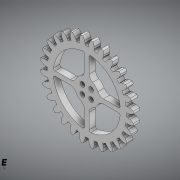
# Autodesk Inventor part: m2z28
Saved by Autodesk Inventor 2020 (Build 240168000, 168)
## iProperties
Created: 2019-12-19
Part Number: m2z28
Material: 一般
Document SubType Name: Modeling
Designer: hamaa
Density: 1 g/cm^3
Appearance: 既定
Author: hamaa
Autodesk Inventor part; units mm, degrees
(part 1 of 2)
ref_plane "YZ Plane" through (0, 0, 0) normal (1, 0, 0) x (0, 1, 0)
ref_plane "XZ Plane" through (0, 0, 0) normal (0, 1, 0) x (-1, 0, 0)
ref_plane "XY Plane" through (0, 0, 0) normal (0, 0, 1) x (1, 0, 0)
sketch "スケッチ1" plane through (0, 0, 0) normal (0, 0, 1) x (1, 0, 0)
  arc A0 (149.6341, 131.6283) -> (149.5837, 131.2892) centre (152.0661, 131.0939) ccw
  arc A1 (149.9967, 132.7811) -> (149.6341, 131.6283) centre (156.3128, 130.1609) ccw
  arc A2 (151.1315, 134.8845) -> (149.9967, 132.7811) centre (160.8866, 128.2635) ccw
  arc A3 (143.6803, 131.213) -> (143.7067, 130.8712) centre (146.1702, 131.2332) ccw
  arc A4 (143.7773, 132.4176) -> (143.6803, 131.213) centre (150.5181, 131.2686) ccw
  arc A5 (144.4157, 134.7208) -> (143.7773, 132.4176) centre (155.3994, 130.4365) ccw
  arc A6 (137.9682, 129.4833) -> (138.07, 129.156) centre (140.3912, 130.0571) ccw
  arc A7 (137.7948, 130.6793) -> (137.9682, 129.4833) centre (144.6222, 131.0591) ccw
  arc A8 (137.9046, 133.0668) -> (137.7948, 130.6793) centre (149.5663, 131.334) ccw
  arc A9 (132.7843, 126.5259) -> (132.9563, 126.2295) centre (135.0188, 127.6245) ccw
  arc A10 (132.349, 127.6534) -> (132.7843, 126.5259) centre (138.9208, 129.5428) ccw
  arc A11 (131.9248, 130.0054) -> (132.349, 127.6534) centre (143.6798, 130.9111) ccw
  arc A12 (128.3884, 122.4892) -> (128.6221, 122.2384) centre (130.3224, 124.0574) ccw
  arc A13 (127.7131, 123.4915) -> (128.3884, 122.4892) centre (133.6997, 126.7959) ccw
  arc A14 (126.7762, 125.6902) -> (127.7131, 123.4915) centre (138.0349, 129.1888) ccw
  arc A15 (125.0009, 117.5754) -> (125.2846, 117.383) centre (126.5375, 119.5348) ccw
  arc A16 (124.1196, 118.4024) -> (125.0009, 117.5754) centre (129.2208, 122.9561) ccw
  arc A17 (122.7169, 120.3375) -> (124.1196, 118.4024) centre (132.9148, 126.2537) ccw
  arc A18 (122.7918, 112.0311) -> (123.1112, 111.9066) centre (123.8539, 114.2832) ccw
  arc A19 (121.7486, 112.6412) -> (122.7918, 112.0311) centre (125.7086, 118.2159) ccw
  arc A20 (119.9505, 114.2156) -> (121.7486, 112.6412) centre (128.5762, 122.2528) ccw
  arc A21 (121.8719, 106.1342) -> (122.2109, 106.0839) centre (122.4062, 108.5662) ccw
  arc A22 (120.719, 106.4969) -> (121.8719, 106.1342) centre (123.3392, 112.813) ccw
  arc A23 (118.6156, 107.6317) -> (120.719, 106.4969) centre (125.2366, 117.3868) ccw
  arc A24 (122.2871, 100.1805) -> (122.6289, 100.2069) centre (122.2669, 102.6704) ccw
  arc A25 (121.0825, 100.2775) -> (122.2871, 100.1805) centre (122.2315, 107.0183) ccw
  arc A26 (118.7793, 100.9159) -> (121.0825, 100.2775) centre (123.0636, 111.8996) ccw
  arc A27 (124.0168, 94.4684) -> (124.3441, 94.5702) centre (123.443, 96.8914) ccw
  arc A28 (122.8208, 94.2949) -> (124.0168, 94.4684) centre (122.441, 101.1224) ccw
  arc A29 (120.4333, 94.4048) -> (122.8208, 94.2949) centre (122.1661, 106.0665) ccw
  arc A30 (126.9742, 89.2845) -> (127.2707, 89.4565) centre (125.8756, 91.519) ccw
  arc A31 (125.8467, 88.8492) -> (126.9742, 89.2845) centre (123.9573, 95.421) ccw
  arc A32 (123.4947, 88.425) -> (125.8467, 88.8492) centre (122.589, 100.1799) ccw
  arc A33 (131.0109, 84.8886) -> (131.2617, 85.1223) centre (129.4427, 86.8226) ccw
  arc A34 (130.0086, 84.2133) -> (131.0109, 84.8886) centre (126.7042, 90.1999) ccw
  arc A35 (127.8099, 83.2764) -> (130.0086, 84.2133) centre (124.3113, 94.5351) ccw
  arc A36 (135.9247, 81.5011) -> (136.1172, 81.7848) centre (133.9654, 83.0377) ccw
  arc A37 (135.0977, 80.6198) -> (135.9247, 81.5011) centre (130.544, 85.721) ccw
  arc A38 (133.1627, 79.2171) -> (135.0977, 80.6198) centre (127.2464, 89.415) ccw
  arc A39 (141.469, 79.292) -> (141.5935, 79.6114) centre (139.2169, 80.3541) ccw
  arc A40 (140.8589, 78.2488) -> (141.469, 79.292) centre (135.2842, 82.2087) ccw
  arc A41 (139.2845, 76.4506) -> (140.8589, 78.2488) centre (131.2473, 85.0764) ccw
  arc A42 (147.3659, 78.372) -> (147.4162, 78.7111) centre (144.9339, 78.9064) ccw
  arc A43 (147.0032, 77.2192) -> (147.3659, 78.372) centre (140.6871, 79.8394) ccw
  arc A44 (145.8684, 75.1158) -> (147.0032, 77.2192) centre (136.1133, 81.7368) ccw
  arc A45 (153.3196, 78.7873) -> (153.2932, 79.1291) centre (150.8297, 78.7671) ccw
  arc A46 (153.2226, 77.5827) -> (153.3196, 78.7873) centre (146.4818, 78.7317) ccw
  arc A47 (152.5843, 75.2795) -> (153.2226, 77.5827) centre (141.6005, 79.5638) ccw
  arc A48 (159.0317, 80.517) -> (158.9299, 80.8443) centre (156.6087, 79.9432) ccw
  arc A49 (159.2052, 79.321) -> (159.0317, 80.517) centre (152.3777, 78.9412) ccw
  arc A50 (159.0953, 76.9335) -> (159.2052, 79.321) centre (147.4336, 78.6663) ccw
  arc A51 (164.2156, 83.4744) -> (164.0436, 83.7708) centre (161.9811, 82.3758) ccw
  arc A52 (164.6509, 82.3469) -> (164.2156, 83.4744) centre (158.0791, 80.4575) ccw
  arc A53 (165.0751, 79.9949) -> (164.6509, 82.3469) centre (153.3202, 79.0892) ccw
  arc A54 (168.6116, 87.5111) -> (168.3778, 87.7619) centre (166.6775, 85.9429) ccw
  arc A55 (169.2868, 86.5088) -> (168.6116, 87.5111) centre (163.3002, 83.2044) ccw
  arc A56 (170.2237, 84.3101) -> (169.2868, 86.5088) centre (158.965, 80.8115) ccw
  arc A57 (171.999, 92.4249) -> (171.7153, 92.6173) centre (170.4624, 90.4655) ccw
  arc A58 (172.8803, 91.5979) -> (171.999, 92.4249) centre (167.7792, 87.0442) ccw
  arc A59 (174.283, 89.6628) -> (172.8803, 91.5979) centre (164.0851, 83.7466) ccw
  arc A60 (174.2081, 97.9692) -> (173.8887, 98.0937) centre (173.146, 95.7171) ccw
  arc A61 (175.2514, 97.3591) -> (174.2081, 97.9692) centre (171.2914, 91.7844) ccw
  arc A62 (177.0495, 95.7847) -> (175.2514, 97.3591) centre (168.4237, 87.7475) ccw
  arc A63 (175.1281, 103.8661) -> (174.789, 103.9164) centre (174.5937, 101.4341) ccw
  arc A64 (176.2809, 103.5034) -> (175.1281, 103.8661) centre (173.6607, 97.1873) ccw
  arc A65 (178.3843, 102.3686) -> (176.2809, 103.5034) centre (171.7633, 92.6135) ccw
  arc A66 (174.7128, 109.8198) -> (174.371, 109.7934) centre (174.733, 107.3299) ccw
  arc A67 (175.9175, 109.7228) -> (174.7128, 109.8198) centre (174.7684, 102.982) ccw
  arc A68 (178.2206, 109.0844) -> (175.9175, 109.7228) centre (173.9363, 98.1007) ccw
  arc A69 (172.9831, 115.5319) -> (172.6558, 115.4301) centre (173.5569, 113.1089) ccw
  arc A70 (174.1792, 115.7054) -> (172.9831, 115.5319) centre (174.5589, 108.8779) ccw
  arc A71 (176.5666, 115.5955) -> (174.1792, 115.7054) centre (174.8338, 103.9338) ccw
  arc A72 (170.0257, 120.7158) -> (169.7293, 120.5438) centre (171.1243, 118.4813) ccw
  arc A73 (171.1532, 121.1511) -> (170.0257, 120.7158) centre (173.0426, 114.5793) ccw
  arc A74 (173.5053, 121.5753) -> (171.1532, 121.1511) centre (174.4109, 109.8203) ccw
  arc A75 (165.989, 125.1117) -> (165.7382, 124.878) centre (167.5573, 123.1777) ccw
  arc A76 (166.9913, 125.787) -> (165.989, 125.1117) centre (170.2957, 119.8004) ccw
  arc A77 (169.19, 126.7239) -> (166.9913, 125.787) centre (172.6887, 115.4652) ccw
  arc A78 (161.0752, 128.4992) -> (160.8828, 128.2155) centre (163.0346, 126.9626) ccw
  arc A79 (161.9022, 129.3805) -> (161.0752, 128.4992) centre (166.4559, 124.2793) ccw
  arc A80 (163.8373, 130.7832) -> (161.9022, 129.3805) centre (169.7535, 120.5853) ccw
  arc A81 (155.5309, 130.7083) -> (155.4064, 130.3889) centre (157.7831, 129.6462) ccw
  arc A82 (156.141, 131.7515) -> (155.5309, 130.7083) centre (161.7157, 127.7915) ccw
  arc A83 (157.7155, 133.5497) -> (156.141, 131.7515) centre (165.7526, 124.9239) ccw
  arc A84 (147.4162, 131.2892) -> (147.3659, 131.6283) centre (144.9339, 131.0939) ccw
  arc A85 (147.3659, 131.6283) -> (147.0032, 132.7811) centre (140.6871, 130.1609) ccw
  arc A86 (147.0032, 132.7811) -> (145.8684, 134.8845) centre (136.1133, 128.2635) ccw
  arc A87 (141.5935, 130.3889) -> (141.469, 130.7083) centre (139.2169, 129.6462) ccw
  arc A88 (141.469, 130.7083) -> (140.8589, 131.7515) centre (135.2842, 127.7915) ccw
  arc A89 (140.8589, 131.7515) -> (139.2845, 133.5497) centre (131.2473, 124.9239) ccw
  arc A90 (136.1172, 128.2155) -> (135.9247, 128.4992) centre (133.9654, 126.9626) ccw
  arc A91 (135.9247, 128.4992) -> (135.0977, 129.3805) centre (130.544, 124.2793) ccw
  arc A92 (135.0977, 129.3805) -> (133.1627, 130.7832) centre (127.2464, 120.5853) ccw
  arc A93 (131.2617, 124.878) -> (131.0109, 125.1117) centre (129.4427, 123.1777) ccw
  arc A94 (131.0109, 125.1117) -> (130.0086, 125.787) centre (126.7042, 119.8004) ccw
  arc A95 (130.0086, 125.787) -> (127.8099, 126.7239) centre (124.3113, 115.4652) ccw
  arc A96 (127.2707, 120.5438) -> (126.9742, 120.7158) centre (125.8756, 118.4813) ccw
  arc A97 (126.9742, 120.7158) -> (125.8467, 121.1511) centre (123.9573, 114.5793) ccw
  arc A98 (125.8467, 121.1511) -> (123.4947, 121.5753) centre (122.589, 109.8203) ccw
  arc A99 (124.3441, 115.4301) -> (124.0168, 115.5319) centre (123.443, 113.1089) ccw
  arc A100 (124.0168, 115.5319) -> (122.8208, 115.7054) centre (122.441, 108.8779) ccw
  arc A101 (122.8208, 115.7054) -> (120.4333, 115.5955) centre (122.1661, 103.9338) ccw
  arc A102 (122.6289, 109.7934) -> (122.2871, 109.8198) centre (122.2669, 107.3299) ccw
  arc A103 (122.2871, 109.8198) -> (121.0825, 109.7228) centre (122.2315, 102.982) ccw
  arc A104 (121.0825, 109.7228) -> (118.7793, 109.0844) centre (123.0636, 98.1007) ccw
  arc A105 (122.2109, 103.9164) -> (121.8719, 103.8661) centre (122.4062, 101.4341) ccw
  arc A106 (121.8719, 103.8661) -> (120.719, 103.5034) centre (123.3392, 97.1873) ccw
  arc A107 (120.719, 103.5034) -> (118.6156, 102.3686) centre (125.2366, 92.6135) ccw
  arc A108 (123.1112, 98.0937) -> (122.7918, 97.9692) centre (123.8539, 95.7171) ccw
  arc A109 (122.7918, 97.9692) -> (121.7486, 97.3591) centre (125.7086, 91.7844) ccw
  arc A110 (121.7486, 97.3591) -> (119.9505, 95.7847) centre (128.5762, 87.7475) ccw
  arc A111 (125.2846, 92.6173) -> (125.0009, 92.4249) centre (126.5375, 90.4655) ccw
  arc A112 (125.0009, 92.4249) -> (124.1196, 91.5979) centre (129.2208, 87.0442) ccw
  arc A113 (124.1196, 91.5979) -> (122.7169, 89.6628) centre (132.9148, 83.7466) ccw
  arc A114 (128.6221, 87.7619) -> (128.3884, 87.5111) centre (130.3224, 85.9429) ccw
  arc A115 (128.3884, 87.5111) -> (127.7131, 86.5088) centre (133.6997, 83.2044) ccw
  arc A116 (127.7131, 86.5088) -> (126.7762, 84.3101) centre (138.0349, 80.8115) ccw
  arc A117 (132.9563, 83.7708) -> (132.7843, 83.4744) centre (135.0188, 82.3758) ccw
  arc A118 (132.7843, 83.4744) -> (132.349, 82.3469) centre (138.9208, 80.4575) ccw
  arc A119 (132.349, 82.3469) -> (131.9248, 79.9949) centre (143.6798, 79.0892) ccw
  arc A120 (138.07, 80.8443) -> (137.9682, 80.517) centre (140.3912, 79.9432) ccw
  arc A121 (137.9682, 80.517) -> (137.7948, 79.321) centre (144.6222, 78.9412) ccw
  arc A122 (137.7948, 79.321) -> (137.9046, 76.9335) centre (149.5663, 78.6663) ccw
  arc A123 (143.7067, 79.1291) -> (143.6803, 78.7873) centre (146.1702, 78.7671) ccw
  arc A124 (143.6803, 78.7873) -> (143.7773, 77.5827) centre (150.5181, 78.7317) ccw
  arc A125 (143.7773, 77.5827) -> (144.4157, 75.2795) centre (155.3994, 79.5638) ccw
  arc A126 (149.5837, 78.7111) -> (149.6341, 78.372) centre (152.0661, 78.9064) ccw
  arc A127 (149.6341, 78.372) -> (149.9967, 77.2192) centre (156.3128, 79.8394) ccw
  arc A128 (149.9967, 77.2192) -> (151.1315, 75.1158) centre (160.8866, 81.7368) ccw
  arc A129 (155.4064, 79.6114) -> (155.5309, 79.292) centre (157.7831, 80.3541) ccw
  arc A130 (155.5309, 79.292) -> (156.141, 78.2488) centre (161.7157, 82.2087) ccw
  arc A131 (156.141, 78.2488) -> (157.7155, 76.4506) centre (165.7526, 85.0764) ccw
  arc A132 (160.8828, 81.7848) -> (161.0752, 81.5011) centre (163.0346, 83.0377) ccw
  arc A133 (161.0752, 81.5011) -> (161.9022, 80.6198) centre (166.4559, 85.721) ccw
  arc A134 (161.9022, 80.6198) -> (163.8373, 79.2171) centre (169.7535, 89.415) ccw
  arc A135 (165.7382, 85.1223) -> (165.989, 84.8886) centre (167.5573, 86.8226) ccw
  arc A136 (165.989, 84.8886) -> (166.9913, 84.2133) centre (170.2957, 90.1999) ccw
  arc A137 (166.9913, 84.2133) -> (169.19, 83.2764) centre (172.6887, 94.5351) ccw
  arc A138 (169.7293, 89.4565) -> (170.0257, 89.2845) centre (171.1243, 91.519) ccw
  arc A139 (170.0257, 89.2845) -> (171.1532, 88.8492) centre (173.0426, 95.421) ccw
  arc A140 (171.1532, 88.8492) -> (173.5053, 88.425) centre (174.4109, 100.1799) ccw
  arc A141 (172.6558, 94.5702) -> (172.9831, 94.4684) centre (173.5569, 96.8914) ccw
  arc A142 (172.9831, 94.4684) -> (174.1792, 94.2949) centre (174.5589, 101.1224) ccw
  arc A143 (174.1792, 94.2949) -> (176.5666, 94.4048) centre (174.8338, 106.0665) ccw
  arc A144 (174.371, 100.2069) -> (174.7128, 100.1805) centre (174.733, 102.6704) ccw
  arc A145 (174.7128, 100.1805) -> (175.9175, 100.2775) centre (174.7684, 107.0183) ccw
  arc A146 (175.9175, 100.2775) -> (178.2206, 100.9159) centre (173.9363, 111.8996) ccw
  arc A147 (174.789, 106.0839) -> (175.1281, 106.1342) centre (174.5937, 108.5662) ccw
  arc A148 (175.1281, 106.1342) -> (176.2809, 106.4969) centre (173.6607, 112.813) ccw
  arc A149 (176.2809, 106.4969) -> (178.3843, 107.6317) centre (171.7633, 117.3868) ccw
  arc A150 (173.8887, 111.9066) -> (174.2081, 112.0311) centre (173.146, 114.2832) ccw
  arc A151 (174.2081, 112.0311) -> (175.2514, 112.6412) centre (171.2914, 118.2159) ccw
  arc A152 (175.2514, 112.6412) -> (177.0495, 114.2156) centre (168.4237, 122.2528) ccw
  arc A153 (171.7153, 117.383) -> (171.999, 117.5754) centre (170.4624, 119.5348) ccw
  arc A154 (171.999, 117.5754) -> (172.8803, 118.4024) centre (167.7792, 122.9561) ccw
  arc A155 (172.8803, 118.4024) -> (174.283, 120.3375) centre (164.0851, 126.2537) ccw
  arc A156 (168.3778, 122.2384) -> (168.6116, 122.4892) centre (166.6775, 124.0574) ccw
  arc A157 (168.6116, 122.4892) -> (169.2868, 123.4915) centre (163.3002, 126.7959) ccw
  arc A158 (169.2868, 123.4915) -> (170.2237, 125.6902) centre (158.965, 129.1888) ccw
  arc A159 (164.0436, 126.2295) -> (164.2156, 126.5259) centre (161.9811, 127.6245) ccw
  arc A160 (164.2156, 126.5259) -> (164.6509, 127.6534) centre (158.0791, 129.5428) ccw
  arc A161 (164.6509, 127.6534) -> (165.0751, 130.0054) centre (153.3202, 130.9111) ccw
  arc A162 (158.9299, 129.156) -> (159.0317, 129.4833) centre (156.6087, 130.0571) ccw
  arc A163 (159.0317, 129.4833) -> (159.2052, 130.6793) centre (152.3777, 131.0591) ccw
  arc A164 (159.2052, 130.6793) -> (159.0953, 133.0668) centre (147.4336, 131.334) ccw
  arc A165 (153.2932, 130.8712) -> (153.3196, 131.213) centre (150.8297, 131.2332) ccw
  arc A166 (153.3196, 131.213) -> (153.2226, 132.4176) centre (146.4818, 131.2686) ccw
  arc A167 (153.2226, 132.4176) -> (152.5843, 134.7208) centre (141.6005, 130.4365) ccw
  arc A168 (149.5503, 130.4785) -> (147.4496, 130.4785) centre (148.5, 105.0001) ccw
  arc A169 (143.8545, 130.0734) -> (141.8065, 129.606) centre (148.5, 105.0001) ccw
  arc A170 (138.3916, 128.4111) -> (136.499, 127.4996) centre (148.5, 105.0001) ccw
  arc A171 (133.4357, 125.5748) -> (131.7933, 124.2651) centre (148.5, 105.0001) ccw
  arc A172 (129.2351, 121.7068) -> (127.9253, 120.0645) centre (148.5, 105.0001) ccw
  arc A173 (126.0005, 117.0011) -> (125.089, 115.1085) centre (148.5, 105.0001) ccw
  arc A174 (123.8941, 111.6936) -> (123.4267, 109.6456) centre (148.5, 105.0001) ccw
  arc A175 (123.0216, 106.0505) -> (123.0216, 103.9498) centre (148.5, 105.0001) ccw
  arc A176 (123.4267, 100.3547) -> (123.8941, 98.3067) centre (148.5, 105.0001) ccw
  arc A177 (125.089, 94.8918) -> (126.0005, 92.9992) centre (148.5, 105.0001) ccw
  arc A178 (127.9253, 89.9358) -> (129.2351, 88.2935) centre (148.5, 105.0001) ccw
  arc A179 (131.7933, 85.7352) -> (133.4357, 84.4255) centre (148.5, 105.0001) ccw
  arc A180 (136.499, 82.5007) -> (138.3916, 81.5892) centre (148.5, 105.0001) ccw
  arc A181 (141.8065, 80.3943) -> (143.8545, 79.9269) centre (148.5, 105.0001) ccw
  arc A182 (147.4496, 79.5218) -> (149.5503, 79.5218) centre (148.5, 105.0001) ccw
  arc A183 (153.1454, 79.9269) -> (155.1934, 80.3943) centre (148.5, 105.0001) ccw
  arc A184 (158.6083, 81.5892) -> (160.5009, 82.5007) centre (148.5, 105.0001) ccw
  arc A185 (163.5643, 84.4255) -> (165.2066, 85.7352) centre (148.5, 105.0001) ccw
  arc A186 (167.7649, 88.2935) -> (169.0746, 89.9358) centre (148.5, 105.0001) ccw
  arc A187 (170.9994, 92.9992) -> (171.9109, 94.8918) centre (148.5, 105.0001) ccw
  arc A188 (173.1058, 98.3067) -> (173.5732, 100.3547) centre (148.5, 105.0001) ccw
  arc A189 (173.9783, 103.9498) -> (173.9783, 106.0505) centre (148.5, 105.0001) ccw
  arc A190 (173.5732, 109.6456) -> (173.1058, 111.6936) centre (148.5, 105.0001) ccw
  arc A191 (171.9109, 115.1085) -> (170.9994, 117.0011) centre (148.5, 105.0001) ccw
  arc A192 (169.0746, 120.0645) -> (167.7649, 121.7068) centre (148.5, 105.0001) ccw
  arc A193 (165.2066, 124.2651) -> (163.5643, 125.5748) centre (148.5, 105.0001) ccw
  arc A194 (160.5009, 127.4996) -> (158.6083, 128.4111) centre (148.5, 105.0001) ccw
  arc A195 (155.1934, 129.606) -> (153.1454, 130.0734) centre (148.5, 105.0001) ccw
  arc A196 (145.8684, 134.8845) -> (144.4157, 134.7208) centre (148.5, 105.0001) ccw
  arc A197 (139.2845, 133.5497) -> (137.9046, 133.0668) centre (148.5, 105.0001) ccw
  arc A198 (133.1627, 130.7832) -> (131.9248, 130.0054) centre (148.5, 105.0001) ccw
  arc A199 (127.8099, 126.7239) -> (126.7762, 125.6902) centre (148.5, 105.0001) ccw
  arc A200 (123.4947, 121.5753) -> (122.7169, 120.3375) centre (148.5, 105.0001) ccw
  arc A201 (120.4333, 115.5955) -> (119.9505, 114.2156) centre (148.5, 105.0001) ccw
  arc A202 (118.7793, 109.0844) -> (118.6156, 107.6317) centre (148.5, 105.0001) ccw
  arc A203 (118.6156, 102.3686) -> (118.7793, 100.9159) centre (148.5, 105.0001) ccw
  arc A204 (119.9505, 95.7847) -> (120.4333, 94.4048) centre (148.5, 105.0001) ccw
  arc A205 (122.7169, 89.6628) -> (123.4947, 88.425) centre (148.5, 105.0001) ccw
  arc A206 (126.7762, 84.3101) -> (127.8099, 83.2764) centre (148.5, 105.0001) ccw
  arc A207 (131.9248, 79.9949) -> (133.1627, 79.2171) centre (148.5, 105.0001) ccw
  arc A208 (137.9046, 76.9335) -> (139.2845, 76.4506) centre (148.5, 105.0001) ccw
  arc A209 (144.4157, 75.2795) -> (145.8684, 75.1158) centre (148.5, 105.0001) ccw
  arc A210 (151.1315, 75.1158) -> (152.5843, 75.2795) centre (148.5, 105.0001) ccw
  arc A211 (157.7155, 76.4506) -> (159.0953, 76.9335) centre (148.5, 105.0001) ccw
  arc A212 (163.8373, 79.2171) -> (165.0751, 79.9949) centre (148.5, 105.0001) ccw
  arc A213 (169.19, 83.2764) -> (170.2237, 84.3101) centre (148.5, 105.0001) ccw
  arc A214 (173.5053, 88.425) -> (174.283, 89.6628) centre (148.5, 105.0001) ccw
  arc A215 (176.5666, 94.4048) -> (177.0495, 95.7847) centre (148.5, 105.0001) ccw
  arc A216 (178.2206, 100.9159) -> (178.3843, 102.3686) centre (148.5, 105.0001) ccw
  arc A217 (178.3843, 107.6317) -> (178.2206, 109.0844) centre (148.5, 105.0001) ccw
  arc A218 (177.0495, 114.2156) -> (176.5666, 115.5955) centre (148.5, 105.0001) ccw
  arc A219 (174.283, 120.3375) -> (173.5053, 121.5753) centre (148.5, 105.0001) ccw
  arc A220 (170.2237, 125.6902) -> (169.19, 126.7239) centre (148.5, 105.0001) ccw
  arc A221 (165.0751, 130.0054) -> (163.8373, 130.7832) centre (148.5, 105.0001) ccw
  arc A222 (159.0953, 133.0668) -> (157.7155, 133.5497) centre (148.5, 105.0001) ccw
  arc A223 (152.5843, 134.7208) -> (151.1315, 134.8845) centre (148.5, 105.0001) ccw
  line L0 (149.5503, 130.4785) -> (149.5837, 131.2892)
  line L1 (143.8545, 130.0734) -> (143.7067, 130.8712)
  line L2 (138.3916, 128.4111) -> (138.07, 129.156)
  line L3 (133.4357, 125.5748) -> (132.9563, 126.2295)
  line L4 (129.2351, 121.7068) -> (128.6221, 122.2384)
  line L5 (126.0005, 117.0011) -> (125.2846, 117.383)
  line L6 (123.8941, 111.6936) -> (123.1112, 111.9066)
  line L7 (123.0216, 106.0505) -> (122.2109, 106.0839)
  line L8 (123.4267, 100.3547) -> (122.6289, 100.2069)
  line L9 (125.089, 94.8918) -> (124.3441, 94.5702)
  line L10 (127.9253, 89.9358) -> (127.2707, 89.4565)
  line L11 (131.7933, 85.7352) -> (131.2617, 85.1223)
  line L12 (136.499, 82.5007) -> (136.1172, 81.7848)
  line L13 (141.8065, 80.3943) -> (141.5935, 79.6114)
  line L14 (147.4496, 79.5218) -> (147.4162, 78.7111)
  line L15 (153.1454, 79.9269) -> (153.2932, 79.1291)
  line L16 (158.6083, 81.5892) -> (158.9299, 80.8443)
  line L17 (163.5643, 84.4255) -> (164.0436, 83.7708)
  line L18 (167.7649, 88.2935) -> (168.3778, 87.7619)
  line L19 (170.9994, 92.9992) -> (171.7153, 92.6173)
  line L20 (173.1058, 98.3067) -> (173.8887, 98.0937)
  line L21 (173.9783, 103.9498) -> (174.789, 103.9164)
  line L22 (173.5732, 109.6456) -> (174.371, 109.7934)
  line L23 (171.9109, 115.1085) -> (172.6558, 115.4301)
  line L24 (169.0746, 120.0645) -> (169.7293, 120.5438)
  line L25 (165.2066, 124.2651) -> (165.7382, 124.878)
  line L26 (160.5009, 127.4996) -> (160.8828, 128.2155)
  line L27 (155.1934, 129.606) -> (155.4064, 130.3889)
  line L28 (147.4496, 130.4785) -> (147.4162, 131.2892)
  line L29 (141.8065, 129.606) -> (141.5935, 130.3889)
  line L30 (136.499, 127.4996) -> (136.1172, 128.2155)
  line L31 (131.7933, 124.2651) -> (131.2617, 124.878)
  line L32 (127.9253, 120.0645) -> (127.2707, 120.5438)
  line L33 (125.089, 115.1085) -> (124.3441, 115.4301)
  line L34 (123.4267, 109.6456) -> (122.6289, 109.7934)
  line L35 (123.0216, 103.9498) -> (122.2109, 103.9164)
  line L36 (123.8941, 98.3067) -> (123.1112, 98.0937)
  line L37 (126.0005, 92.9992) -> (125.2846, 92.6173)
  line L38 (129.2351, 88.2935) -> (128.6221, 87.7619)
  line L39 (133.4357, 84.4255) -> (132.9563, 83.7708)
  line L40 (138.3916, 81.5892) -> (138.07, 80.8443)
  line L41 (143.8545, 79.9269) -> (143.7067, 79.1291)
  line L42 (149.5503, 79.5218) -> (149.5837, 78.7111)
  line L43 (155.1934, 80.3943) -> (155.4064, 79.6114)
  line L44 (160.5009, 82.5007) -> (160.8828, 81.7848)
  line L45 (165.2066, 85.7352) -> (165.7382, 85.1223)
  line L46 (169.0746, 89.9358) -> (169.7293, 89.4565)
  line L47 (171.9109, 94.8918) -> (172.6558, 94.5702)
  line L48 (173.5732, 100.3547) -> (174.371, 100.2069)
  line L49 (173.9783, 106.0505) -> (174.789, 106.0839)
  line L50 (173.1058, 111.6936) -> (173.8887, 111.9066)
  line L51 (170.9994, 117.0011) -> (171.7153, 117.383)
  line L52 (167.7649, 121.7068) -> (168.3778, 122.2384)
  line L53 (163.5643, 125.5748) -> (164.0436, 126.2295)
  line L54 (158.6083, 128.4111) -> (158.9299, 129.156)
  line L55 (153.1454, 130.0734) -> (153.2932, 130.8712)
  line L56 (116.5, 105) -> (180.5, 105)
  line L57 (148.5, 73) -> (148.5, 137)
  line L58 (198.5, 135.0001) -> (268.5, 135.0001)
  line L59 (198.5, 127.0001) -> (268.5, 127.0001)
  line L60 (198.5, 119.0001) -> (268.5, 119.0001)
  line L61 (198.5, 111.0001) -> (268.5, 111.0001)
  line L62 (198.5, 103.0001) -> (268.5, 103.0001)
  line L63 (198.5, 95.0001) -> (268.5, 95.0001)
  line L64 (198.5, 87.0001) -> (268.5, 87.0001)
  line L65 (198.5, 79.0001) -> (268.5, 79.0001)
  line L66 (198.5, 71.0001) -> (268.5, 71.0001)
  line L67 (198.5, 63.0001) -> (268.5, 63.0001)
  line L68 (198.5, 55.0001) -> (268.5, 55.0001)
  line L69 (198.5, 47.0001) -> (268.5, 47.0001)
  line L70 (198.5, 39.0001) -> (268.5, 39.0001)
  line L71 (198.5, 135.0001) -> (198.5, 39.0001)
  line L72 (268.5, 135.0001) -> (268.5, 39.0001)
  line L73 (233.5, 127.0001) -> (233.5, 39.0001)
  point P0 (0, 0)
  point P1 (204.5, 129)
  point P2 (207, 121)
  point P3 (207, 113)
  point P4 (204.5, 105)
  point P5 (207, 97)
  point P6 (202, 89)
  point P7 (204.5, 81)
  point P8 (204.5, 73)
  point P9 (204.5, 65)
  point P10 (207, 57)
  point P11 (207, 49)
  point P12 (204.5, 41)
  point P13 (234.5, 121)
  point P14 (249.5, 113)
  point P15 (250.75, 105)
  point P16 (247, 97)
  point P17 (249.5, 89)
  point P18 (243.25, 81)
  point P19 (249.5, 73)
  point P20 (249.5, 65)
  point P21 (244.5, 57)
  point P22 (252, 49)
  point P23 (252, 41)
  point P24 (149.5, 150.5)
  point P25 (149.5, 144.5)
  point P26 (165.6875, 150.5)
  point P27 (168.875, 144.5)
  constraints: 336 point on circle, 168 centre point, 165 equal radius, 144 end point, 112 tangent, 41 parallel, 30 horizontal, 16 perpendicular, 2 horizontal alignment, 2 midpoint, 2 vertical alignment, 219 other
extrude "押し出し1" add sketch "スケッチ1" along normal blind 4 contours A1 A2 A223 A167 A166 A165 L55 A195 L27 A81 A82 A83 A222 A164 A163 A162 L54 A194 L26 A78 A79 A80 A221 A161 A160 A159 L53 A193 L25 A75 A76 A77 A220 A158 A157 A156 L52 A192 L24 A72 A73 A74 A219 A155 A154 A153 L51 A191 L23 A69 A70 A71 A218 A152 A151 A150 L50 A190 L22 A66 A67 A68 A217 A149 A148 A147 L49 A189 L56 L57 A168 L0 A0 | L57 L56 A175 L7 A21 A22 A23 A202 A104 A103 A102 L34 A174 L6 A18 A19 A20 A201 A101 A100 A99 L33 A173 L5 A15 A16 A17 A200 A98 A97 A96 L32 A172 L4 A12 A13 A14 A199 A95 A94 A93 L31 A171 L3 A9 A10 A11 A198 A92 A91 A90 L30 A170 L2 A6 A7 A8 A197 A89 A88 A87 L29 A169 L1 A3 A4 A5 A196 A86 A85 A84 L28 A168 | L57 A182 L14 A42 A43 A44 A209 A125 A124 A123 L41 A181 L13 A39 A40 A41 A208 A122 A121 A120 L40 A180 L12 A36 A37 A38 A207 A119 A118 A117 L39 A179 L11 A33 A34 A35 A206 A116 A115 A114 L38 A178 L10 A30 A31 A32 A205 A113 A112 A111 L37 A177 L9 A27 A28 A29 A204 A110 A109 A108 L36 A176 L8 A24 A25 A26 A203 A107 A106 A105 L35 A175 L56 | L56 A189 L21 A63 A64 A65 A216 A146 A145 A144 L48 A188 L20 A60 A61 A62 A215 A143 A142 A141 L47 A187 L19 A57 A58 A59 A214 A140 A139 A138 L46 A186 L18 A54 A55 A56 A213 A137 A136 A135 L45 A185 L17 A51 A52 A53 A212 A134 A133 A132 L44 A184 L16 A48 A49 A50 A211 A131 A130 A129 L43 A183 L15 A45 A46 A47 A210 A128 A127 A126 L42 A182 L57
sketch "スケッチ2" plane through (0, 0, 4) normal (0, 0, 1) x (1, 0, 0)
  arc A0 (147.4162, 131.2892) -> (147.3659, 131.6283) centre (144.9339, 131.0939) ccw projected
  arc A1 (147.3659, 131.6283) -> (147.0032, 132.7811) centre (140.6871, 130.1609) ccw projected
  arc A2 (147.0032, 132.7811) -> (145.8684, 134.8845) centre (136.1133, 128.2635) ccw projected
  arc A3 (145.8684, 134.8845) -> (144.4157, 134.7208) centre (148.5, 105.0001) ccw projected
  arc A4 (144.4157, 134.7208) -> (143.7773, 132.4176) centre (155.3994, 130.4365) ccw projected
  arc A5 (143.7773, 132.4176) -> (143.6803, 131.213) centre (150.5181, 131.2686) ccw projected
  arc A6 (143.6803, 131.213) -> (143.7067, 130.8712) centre (146.1702, 131.2332) ccw projected
  line L0 (143.7067, 130.8712) -> (143.8545, 130.0734) projected
  arc A7 (143.8545, 130.0734) -> (141.8065, 129.606) centre (148.5, 105.0001) ccw projected
  line L1 (141.8065, 129.606) -> (141.5935, 130.3889) projected
  arc A8 (141.5935, 130.3889) -> (141.469, 130.7083) centre (139.2169, 129.6462) ccw projected
  arc A9 (141.469, 130.7083) -> (140.8589, 131.7515) centre (135.2842, 127.7915) ccw projected
  arc A10 (140.8589, 131.7515) -> (139.2845, 133.5497) centre (131.2473, 124.9239) ccw projected
  arc A11 (139.2845, 133.5497) -> (137.9046, 133.0668) centre (148.5, 105.0001) ccw projected
  arc A12 (137.9046, 133.0668) -> (137.7948, 130.6793) centre (149.5663, 131.334) ccw projected
  arc A13 (137.7948, 130.6793) -> (137.9682, 129.4833) centre (144.6222, 131.0591) ccw projected
  arc A14 (137.9682, 129.4833) -> (138.07, 129.156) centre (140.3912, 130.0571) ccw projected
  line L2 (138.07, 129.156) -> (138.3916, 128.4111) projected
  arc A15 (138.3916, 128.4111) -> (136.499, 127.4996) centre (148.5, 105.0001) ccw projected
  line L3 (136.499, 127.4996) -> (136.1172, 128.2155) projected
  arc A16 (136.1172, 128.2155) -> (135.9247, 128.4992) centre (133.9654, 126.9626) ccw projected
  arc A17 (135.9247, 128.4992) -> (135.0977, 129.3805) centre (130.544, 124.2793) ccw projected
  arc A18 (135.0977, 129.3805) -> (133.1627, 130.7832) centre (127.2464, 120.5853) ccw projected
  arc A19 (133.1627, 130.7832) -> (131.9248, 130.0054) centre (148.5, 105.0001) ccw projected
  arc A20 (131.9248, 130.0054) -> (132.349, 127.6534) centre (143.6798, 130.9111) ccw projected
  arc A21 (132.349, 127.6534) -> (132.7843, 126.5259) centre (138.9208, 129.5428) ccw projected
  arc A22 (132.7843, 126.5259) -> (132.9563, 126.2295) centre (135.0188, 127.6245) ccw projected
  line L4 (132.9563, 126.2295) -> (133.4357, 125.5748) projected
  arc A23 (133.4357, 125.5748) -> (131.7933, 124.2651) centre (148.5, 105.0001) ccw projected
  line L5 (131.7933, 124.2651) -> (131.2617, 124.878) projected
  arc A24 (131.2617, 124.878) -> (131.0109, 125.1117) centre (129.4427, 123.1777) ccw projected
  arc A25 (131.0109, 125.1117) -> (130.0086, 125.787) centre (126.7042, 119.8004) ccw projected
  arc A26 (130.0086, 125.787) -> (127.8099, 126.7239) centre (124.3113, 115.4652) ccw projected
  arc A27 (127.8099, 126.7239) -> (126.7762, 125.6902) centre (148.5, 105.0001) ccw projected
  arc A28 (126.7762, 125.6902) -> (127.7131, 123.4915) centre (138.0349, 129.1888) ccw projected
  arc A29 (127.7131, 123.4915) -> (128.3884, 122.4892) centre (133.6997, 126.7959) ccw projected
  arc A30 (128.3884, 122.4892) -> (128.6221, 122.2384) centre (130.3224, 124.0574) ccw projected
  line L6 (128.6221, 122.2384) -> (129.2351, 121.7068) projected
  arc A31 (129.2351, 121.7068) -> (127.9253, 120.0645) centre (148.5, 105.0001) ccw projected
  line L7 (127.9253, 120.0645) -> (127.2707, 120.5438) projected
  arc A32 (127.2707, 120.5438) -> (126.9742, 120.7158) centre (125.8756, 118.4813) ccw projected
  arc A33 (126.9742, 120.7158) -> (125.8467, 121.1511) centre (123.9573, 114.5793) ccw projected
  arc A34 (125.8467, 121.1511) -> (123.4947, 121.5753) centre (122.589, 109.8203) ccw projected
  arc A35 (123.4947, 121.5753) -> (122.7169, 120.3375) centre (148.5, 105.0001) ccw projected
  arc A36 (122.7169, 120.3375) -> (124.1196, 118.4024) centre (132.9148, 126.2537) ccw projected
  arc A37 (124.1196, 118.4024) -> (125.0009, 117.5754) centre (129.2208, 122.9561) ccw projected
  arc A38 (125.0009, 117.5754) -> (125.2846, 117.383) centre (126.5375, 119.5348) ccw projected
  line L8 (125.2846, 117.383) -> (126.0005, 117.0011) projected
  arc A39 (126.0005, 117.0011) -> (125.089, 115.1085) centre (148.5, 105.0001) ccw projected
  line L9 (125.089, 115.1085) -> (124.3441, 115.4301) projected
  arc A40 (124.3441, 115.4301) -> (124.0168, 115.5319) centre (123.443, 113.1089) ccw projected
  arc A41 (124.0168, 115.5319) -> (122.8208, 115.7054) centre (122.441, 108.8779) ccw projected
  arc A42 (122.8208, 115.7054) -> (120.4333, 115.5955) centre (122.1661, 103.9338) ccw projected
  arc A43 (120.4333, 115.5955) -> (119.9505, 114.2156) centre (148.5, 105.0001) ccw projected
  arc A44 (119.9505, 114.2156) -> (121.7486, 112.6412) centre (128.5762, 122.2528) ccw projected
  arc A45 (121.7486, 112.6412) -> (122.7918, 112.0311) centre (125.7086, 118.2159) ccw projected
  arc A46 (122.7918, 112.0311) -> (123.1112, 111.9066) centre (123.8539, 114.2832) ccw projected
  line L10 (123.1112, 111.9066) -> (123.8941, 111.6936) projected
  arc A47 (123.8941, 111.6936) -> (123.4267, 109.6456) centre (148.5, 105.0001) ccw projected
  line L11 (123.4267, 109.6456) -> (122.6289, 109.7934) projected
  arc A48 (122.6289, 109.7934) -> (122.2871, 109.8198) centre (122.2669, 107.3299) ccw projected
  arc A49 (122.2871, 109.8198) -> (121.0825, 109.7228) centre (122.2315, 102.982) ccw projected
  arc A50 (121.0825, 109.7228) -> (118.7793, 109.0844) centre (123.0636, 98.1007) ccw projected
  arc A51 (118.7793, 109.0844) -> (118.6156, 107.6317) centre (148.5, 105.0001) ccw projected
  arc A52 (118.6156, 107.6317) -> (120.719, 106.4969) centre (125.2366, 117.3868) ccw projected
  arc A53 (120.719, 106.4969) -> (121.8719, 106.1342) centre (123.3392, 112.813) ccw projected
  arc A54 (121.8719, 106.1342) -> (122.2109, 106.0839) centre (122.4062, 108.5662) ccw projected
  line L12 (122.2109, 106.0839) -> (123.0216, 106.0505) projected
  arc A55 (123.0216, 106.0505) -> (123.0216, 103.9498) centre (148.5, 105.0001) ccw projected
  line L13 (123.0216, 103.9498) -> (122.2109, 103.9164) projected
  arc A56 (122.2109, 103.9164) -> (121.8719, 103.8661) centre (122.4062, 101.4341) ccw projected
  arc A57 (121.8719, 103.8661) -> (120.719, 103.5034) centre (123.3392, 97.1873) ccw projected
  arc A58 (120.719, 103.5034) -> (118.6156, 102.3686) centre (125.2366, 92.6135) ccw projected
  arc A59 (118.6156, 102.3686) -> (118.7793, 100.9159) centre (148.5, 105.0001) ccw projected
  arc A60 (118.7793, 100.9159) -> (121.0825, 100.2775) centre (123.0636, 111.8996) ccw projected
  arc A61 (121.0825, 100.2775) -> (122.2871, 100.1805) centre (122.2315, 107.0183) ccw projected
  arc A62 (122.2871, 100.1805) -> (122.6289, 100.2069) centre (122.2669, 102.6704) ccw projected
  line L14 (122.6289, 100.2069) -> (123.4267, 100.3547) projected
  arc A63 (123.4267, 100.3547) -> (123.8941, 98.3067) centre (148.5, 105.0001) ccw projected
  line L15 (123.8941, 98.3067) -> (123.1112, 98.0937) projected
  arc A64 (123.1112, 98.0937) -> (122.7918, 97.9692) centre (123.8539, 95.7171) ccw projected
  arc A65 (122.7918, 97.9692) -> (121.7486, 97.3591) centre (125.7086, 91.7844) ccw projected
  arc A66 (121.7486, 97.3591) -> (119.9505, 95.7847) centre (128.5762, 87.7475) ccw projected
  arc A67 (119.9505, 95.7847) -> (120.4333, 94.4048) centre (148.5, 105.0001) ccw projected
  arc A68 (120.4333, 94.4048) -> (122.8208, 94.2949) centre (122.1661, 106.0665) ccw projected
  arc A69 (122.8208, 94.2949) -> (124.0168, 94.4684) centre (122.441, 101.1224) ccw projected
  arc A70 (124.0168, 94.4684) -> (124.3441, 94.5702) centre (123.443, 96.8914) ccw projected
  line L16 (124.3441, 94.5702) -> (125.089, 94.8918) projected
  arc A71 (125.089, 94.8918) -> (126.0005, 92.9992) centre (148.5, 105.0001) ccw projected
  line L17 (126.0005, 92.9992) -> (125.2846, 92.6173) projected
  arc A72 (125.2846, 92.6173) -> (125.0009, 92.4249) centre (126.5375, 90.4655) ccw projected
  arc A73 (125.0009, 92.4249) -> (124.1196, 91.5979) centre (129.2208, 87.0442) ccw projected
  arc A74 (124.1196, 91.5979) -> (122.7169, 89.6628) centre (132.9148, 83.7466) ccw projected
  arc A75 (122.7169, 89.6628) -> (123.4947, 88.425) centre (148.5, 105.0001) ccw projected
  arc A76 (123.4947, 88.425) -> (125.8467, 88.8492) centre (122.589, 100.1799) ccw projected
  arc A77 (125.8467, 88.8492) -> (126.9742, 89.2845) centre (123.9573, 95.421) ccw projected
  arc A78 (126.9742, 89.2845) -> (127.2707, 89.4565) centre (125.8756, 91.519) ccw projected
  line L18 (127.2707, 89.4565) -> (127.9253, 89.9358) projected
  arc A79 (127.9253, 89.9358) -> (129.2351, 88.2935) centre (148.5, 105.0001) ccw projected
  line L19 (129.2351, 88.2935) -> (128.6221, 87.7619) projected
  arc A80 (128.6221, 87.7619) -> (128.3884, 87.5111) centre (130.3224, 85.9429) ccw projected
  arc A81 (128.3884, 87.5111) -> (127.7131, 86.5088) centre (133.6997, 83.2044) ccw projected
  arc A82 (127.7131, 86.5088) -> (126.7762, 84.3101) centre (138.0349, 80.8115) ccw projected
  arc A83 (126.7762, 84.3101) -> (127.8099, 83.2764) centre (148.5, 105.0001) ccw projected
  arc A84 (127.8099, 83.2764) -> (130.0086, 84.2133) centre (124.3113, 94.5351) ccw projected
  arc A85 (130.0086, 84.2133) -> (131.0109, 84.8886) centre (126.7042, 90.1999) ccw projected
  arc A86 (131.0109, 84.8886) -> (131.2617, 85.1223) centre (129.4427, 86.8226) ccw projected
  line L20 (131.2617, 85.1223) -> (131.7933, 85.7352) projected
  arc A87 (131.7933, 85.7352) -> (133.4357, 84.4255) centre (148.5, 105.0001) ccw projected
  line L21 (133.4357, 84.4255) -> (132.9563, 83.7708) projected
  arc A88 (132.9563, 83.7708) -> (132.7843, 83.4744) centre (135.0188, 82.3758) ccw projected
  arc A89 (132.7843, 83.4744) -> (132.349, 82.3469) centre (138.9208, 80.4575) ccw projected
  arc A90 (132.349, 82.3469) -> (131.9248, 79.9949) centre (143.6798, 79.0892) ccw projected
  arc A91 (131.9248, 79.9949) -> (133.1627, 79.2171) centre (148.5, 105.0001) ccw projected
  arc A92 (133.1627, 79.2171) -> (135.0977, 80.6198) centre (127.2464, 89.415) ccw projected
  arc A93 (135.0977, 80.6198) -> (135.9247, 81.5011) centre (130.544, 85.721) ccw projected
  arc A94 (135.9247, 81.5011) -> (136.1172, 81.7848) centre (133.9654, 83.0377) ccw projected
  line L22 (136.1172, 81.7848) -> (136.499, 82.5007) projected
  arc A95 (136.499, 82.5007) -> (138.3916, 81.5892) centre (148.5, 105.0001) ccw projected
  line L23 (138.3916, 81.5892) -> (138.07, 80.8443) projected
  arc A96 (138.07, 80.8443) -> (137.9682, 80.517) centre (140.3912, 79.9432) ccw projected
  arc A97 (137.9682, 80.517) -> (137.7948, 79.321) centre (144.6222, 78.9412) ccw projected
  arc A98 (137.7948, 79.321) -> (137.9046, 76.9335) centre (149.5663, 78.6663) ccw projected
  arc A99 (137.9046, 76.9335) -> (139.2845, 76.4506) centre (148.5, 105.0001) ccw projected
  arc A100 (139.2845, 76.4506) -> (140.8589, 78.2488) centre (131.2473, 85.0764) ccw projected
  arc A101 (140.8589, 78.2488) -> (141.469, 79.292) centre (135.2842, 82.2087) ccw projected
  arc A102 (141.469, 79.292) -> (141.5935, 79.6114) centre (139.2169, 80.3541) ccw projected
  line L24 (141.5935, 79.6114) -> (141.8065, 80.3943) projected
  arc A103 (141.8065, 80.3943) -> (143.8545, 79.9269) centre (148.5, 105.0001) ccw projected
  line L25 (143.8545, 79.9269) -> (143.7067, 79.1291) projected
  arc A104 (143.7067, 79.1291) -> (143.6803, 78.7873) centre (146.1702, 78.7671) ccw projected
  arc A105 (143.6803, 78.7873) -> (143.7773, 77.5827) centre (150.5181, 78.7317) ccw projected
  arc A106 (143.7773, 77.5827) -> (144.4157, 75.2795) centre (155.3994, 79.5638) ccw projected
  arc A107 (144.4157, 75.2795) -> (145.8684, 75.1158) centre (148.5, 105.0001) ccw projected
  arc A108 (145.8684, 75.1158) -> (147.0032, 77.2192) centre (136.1133, 81.7368) ccw projected
  arc A109 (147.0032, 77.2192) -> (147.3659, 78.372) centre (140.6871, 79.8394) ccw projected
  arc A110 (147.3659, 78.372) -> (147.4162, 78.7111) centre (144.9339, 78.9064) ccw projected
  line L26 (147.4162, 78.7111) -> (147.4496, 79.5218) projected
  arc A111 (147.4496, 79.5218) -> (149.5503, 79.5218) centre (148.5, 105.0001) ccw projected
  line L27 (149.5503, 79.5218) -> (149.5837, 78.7111) projected
  arc A112 (149.5837, 78.7111) -> (149.6341, 78.372) centre (152.0661, 78.9064) ccw projected
  arc A113 (149.6341, 78.372) -> (149.9967, 77.2192) centre (156.3128, 79.8394) ccw projected
  arc A114 (149.9967, 77.2192) -> (151.1315, 75.1158) centre (160.8866, 81.7368) ccw projected
  arc A115 (151.1315, 75.1158) -> (152.5843, 75.2795) centre (148.5, 105.0001) ccw projected
  arc A116 (152.5843, 75.2795) -> (153.2226, 77.5827) centre (141.6005, 79.5638) ccw projected
  arc A117 (153.2226, 77.5827) -> (153.3196, 78.7873) centre (146.4818, 78.7317) ccw projected
  arc A118 (153.3196, 78.7873) -> (153.2932, 79.1291) centre (150.8297, 78.7671) ccw projected
  line L28 (153.2932, 79.1291) -> (153.1454, 79.9269) projected
  arc A119 (153.1454, 79.9269) -> (155.1934, 80.3943) centre (148.5, 105.0001) ccw projected
  line L29 (155.1934, 80.3943) -> (155.4064, 79.6114) projected
  arc A120 (155.4064, 79.6114) -> (155.5309, 79.292) centre (157.7831, 80.3541) ccw projected
  arc A121 (155.5309, 79.292) -> (156.141, 78.2488) centre (161.7157, 82.2087) ccw projected
  arc A122 (156.141, 78.2488) -> (157.7155, 76.4506) centre (165.7526, 85.0764) ccw projected
  arc A123 (157.7155, 76.4506) -> (159.0953, 76.9335) centre (148.5, 105.0001) ccw projected
  arc A124 (159.0953, 76.9335) -> (159.2052, 79.321) centre (147.4336, 78.6663) ccw projected
  arc A125 (159.2052, 79.321) -> (159.0317, 80.517) centre (152.3777, 78.9412) ccw projected
  arc A126 (159.0317, 80.517) -> (158.9299, 80.8443) centre (156.6087, 79.9432) ccw projected
  line L30 (158.9299, 80.8443) -> (158.6083, 81.5892) projected
  arc A127 (158.6083, 81.5892) -> (160.5009, 82.5007) centre (148.5, 105.0001) ccw projected
  line L31 (160.5009, 82.5007) -> (160.8828, 81.7848) projected
  arc A128 (160.8828, 81.7848) -> (161.0752, 81.5011) centre (163.0346, 83.0377) ccw projected
  arc A129 (161.0752, 81.5011) -> (161.9022, 80.6198) centre (166.4559, 85.721) ccw projected
  arc A130 (161.9022, 80.6198) -> (163.8373, 79.2171) centre (169.7535, 89.415) ccw projected
  arc A131 (163.8373, 79.2171) -> (165.0751, 79.9949) centre (148.5, 105.0001) ccw projected
  arc A132 (165.0751, 79.9949) -> (164.6509, 82.3469) centre (153.3202, 79.0892) ccw projected
  arc A133 (164.6509, 82.3469) -> (164.2156, 83.4744) centre (158.0791, 80.4575) ccw projected
  arc A134 (164.2156, 83.4744) -> (164.0436, 83.7708) centre (161.9811, 82.3758) ccw projected
  line L32 (164.0436, 83.7708) -> (163.5643, 84.4255) projected
  arc A135 (163.5643, 84.4255) -> (165.2066, 85.7352) centre (148.5, 105.0001) ccw projected
  line L33 (165.2066, 85.7352) -> (165.7382, 85.1223) projected
  arc A136 (165.7382, 85.1223) -> (165.989, 84.8886) centre (167.5573, 86.8226) ccw projected
  arc A137 (165.989, 84.8886) -> (166.9913, 84.2133) centre (170.2957, 90.1999) ccw projected
  arc A138 (166.9913, 84.2133) -> (169.19, 83.2764) centre (172.6887, 94.5351) ccw projected
  arc A139 (169.19, 83.2764) -> (170.2237, 84.3101) centre (148.5, 105.0001) ccw projected
  arc A140 (170.2237, 84.3101) -> (169.2868, 86.5088) centre (158.965, 80.8115) ccw projected
  arc A141 (169.2868, 86.5088) -> (168.6116, 87.5111) centre (163.3002, 83.2044) ccw projected
  arc A142 (168.6116, 87.5111) -> (168.3778, 87.7619) centre (166.6775, 85.9429) ccw projected
  line L34 (168.3778, 87.7619) -> (167.7649, 88.2935) projected
  arc A143 (167.7649, 88.2935) -> (169.0746, 89.9358) centre (148.5, 105.0001) ccw projected
  line L35 (169.0746, 89.9358) -> (169.7293, 89.4565) projected
  arc A144 (169.7293, 89.4565) -> (170.0257, 89.2845) centre (171.1243, 91.519) ccw projected
  arc A145 (170.0257, 89.2845) -> (171.1532, 88.8492) centre (173.0426, 95.421) ccw projected
  arc A146 (171.1532, 88.8492) -> (173.5053, 88.425) centre (174.4109, 100.1799) ccw projected
  arc A147 (173.5053, 88.425) -> (174.283, 89.6628) centre (148.5, 105.0001) ccw projected
  arc A148 (174.283, 89.6628) -> (172.8803, 91.5979) centre (164.0851, 83.7466) ccw projected
  arc A149 (172.8803, 91.5979) -> (171.999, 92.4249) centre (167.7792, 87.0442) ccw projected
  arc A150 (171.999, 92.4249) -> (171.7153, 92.6173) centre (170.4624, 90.4655) ccw projected
  line L36 (171.7153, 92.6173) -> (170.9994, 92.9992) projected
  arc A151 (170.9994, 92.9992) -> (171.9109, 94.8918) centre (148.5, 105.0001) ccw projected
  line L37 (171.9109, 94.8918) -> (172.6558, 94.5702) projected
  arc A152 (172.6558, 94.5702) -> (172.9831, 94.4684) centre (173.5569, 96.8914) ccw projected
  arc A153 (172.9831, 94.4684) -> (174.1792, 94.2949) centre (174.5589, 101.1224) ccw projected
  arc A154 (174.1792, 94.2949) -> (176.5666, 94.4048) centre (174.8338, 106.0665) ccw projected
  arc A155 (176.5666, 94.4048) -> (177.0495, 95.7847) centre (148.5, 105.0001) ccw projected
  arc A156 (177.0495, 95.7847) -> (175.2514, 97.3591) centre (168.4237, 87.7475) ccw projected
  arc A157 (175.2514, 97.3591) -> (174.2081, 97.9692) centre (171.2914, 91.7844) ccw projected
  arc A158 (174.2081, 97.9692) -> (173.8887, 98.0937) centre (173.146, 95.7171) ccw projected
  line L38 (173.8887, 98.0937) -> (173.1058, 98.3067) projected
  arc A159 (173.1058, 98.3067) -> (173.5732, 100.3547) centre (148.5, 105.0001) ccw projected
  line L39 (173.5732, 100.3547) -> (174.371, 100.2069) projected
  arc A160 (174.371, 100.2069) -> (174.7128, 100.1805) centre (174.733, 102.6704) ccw projected
  arc A161 (174.7128, 100.1805) -> (175.9175, 100.2775) centre (174.7684, 107.0183) ccw projected
  arc A162 (175.9175, 100.2775) -> (178.2206, 100.9159) centre (173.9363, 111.8996) ccw projected
  arc A163 (178.2206, 100.9159) -> (178.3843, 102.3686) centre (148.5, 105.0001) ccw projected
  arc A164 (178.3843, 102.3686) -> (176.2809, 103.5034) centre (171.7633, 92.6135) ccw projected
  arc A165 (176.2809, 103.5034) -> (175.1281, 103.8661) centre (173.6607, 97.1873) ccw projected
  arc A166 (175.1281, 103.8661) -> (174.789, 103.9164) centre (174.5937, 101.4341) ccw projected
  line L40 (174.789, 103.9164) -> (173.9783, 103.9498) projected
  arc A167 (173.9783, 103.9498) -> (173.9783, 106.0505) centre (148.5, 105.0001) ccw projected
  line L41 (173.9783, 106.0505) -> (174.789, 106.0839) projected
  arc A168 (174.789, 106.0839) -> (175.1281, 106.1342) centre (174.5937, 108.5662) ccw projected
  arc A169 (175.1281, 106.1342) -> (176.2809, 106.4969) centre (173.6607, 112.813) ccw projected
  arc A170 (176.2809, 106.4969) -> (178.3843, 107.6317) centre (171.7633, 117.3868) ccw projected
  arc A171 (178.3843, 107.6317) -> (178.2206, 109.0844) centre (148.5, 105.0001) ccw projected
  arc A172 (178.2206, 109.0844) -> (175.9175, 109.7228) centre (173.9363, 98.1007) ccw projected
  arc A173 (175.9175, 109.7228) -> (174.7128, 109.8198) centre (174.7684, 102.982) ccw projected
  arc A174 (174.7128, 109.8198) -> (174.371, 109.7934) centre (174.733, 107.3299) ccw projected
  line L42 (174.371, 109.7934) -> (173.5732, 109.6456) projected
  arc A175 (173.5732, 109.6456) -> (173.1058, 111.6936) centre (148.5, 105.0001) ccw projected
  line L43 (173.1058, 111.6936) -> (173.8887, 111.9066) projected
  arc A176 (173.8887, 111.9066) -> (174.2081, 112.0311) centre (173.146, 114.2832) ccw projected
  arc A177 (174.2081, 112.0311) -> (175.2514, 112.6412) centre (171.2914, 118.2159) ccw projected
  arc A178 (175.2514, 112.6412) -> (177.0495, 114.2156) centre (168.4237, 122.2528) ccw projected
  arc A179 (177.0495, 114.2156) -> (176.5666, 115.5955) centre (148.5, 105.0001) ccw projected
  arc A180 (176.5666, 115.5955) -> (174.1792, 115.7054) centre (174.8338, 103.9338) ccw projected
  arc A181 (174.1792, 115.7054) -> (172.9831, 115.5319) centre (174.5589, 108.8779) ccw projected
  arc A182 (172.9831, 115.5319) -> (172.6558, 115.4301) centre (173.5569, 113.1089) ccw projected
  line L44 (172.6558, 115.4301) -> (171.9109, 115.1085) projected
  arc A183 (171.9109, 115.1085) -> (170.9994, 117.0011) centre (148.5, 105.0001) ccw projected
  line L45 (170.9994, 117.0011) -> (171.7153, 117.383) projected
  arc A184 (171.7153, 117.383) -> (171.999, 117.5754) centre (170.4624, 119.5348) ccw projected
  arc A185 (171.999, 117.5754) -> (172.8803, 118.4024) centre (167.7792, 122.9561) ccw projected
  arc A186 (172.8803, 118.4024) -> (174.283, 120.3375) centre (164.0851, 126.2537) ccw projected
  arc A187 (174.283, 120.3375) -> (173.5053, 121.5753) centre (148.5, 105.0001) ccw projected
  arc A188 (173.5053, 121.5753) -> (171.1532, 121.1511) centre (174.4109, 109.8203) ccw projected
  arc A189 (171.1532, 121.1511) -> (170.0257, 120.7158) centre (173.0426, 114.5793) ccw projected
  arc A190 (170.0257, 120.7158) -> (169.7293, 120.5438) centre (171.1243, 118.4813) ccw projected
  line L46 (169.7293, 120.5438) -> (169.0746, 120.0645) projected
  arc A191 (169.0746, 120.0645) -> (167.7649, 121.7068) centre (148.5, 105.0001) ccw projected
  line L47 (167.7649, 121.7068) -> (168.3778, 122.2384) projected
  arc A192 (168.3778, 122.2384) -> (168.6116, 122.4892) centre (166.6775, 124.0574) ccw projected
  arc A193 (168.6116, 122.4892) -> (169.2868, 123.4915) centre (163.3002, 126.7959) ccw projected
  arc A194 (169.2868, 123.4915) -> (170.2237, 125.6902) centre (158.965, 129.1888) ccw projected
  arc A195 (170.2237, 125.6902) -> (169.19, 126.7239) centre (148.5, 105.0001) ccw projected
  arc A196 (169.19, 126.7239) -> (166.9913, 125.787) centre (172.6887, 115.4652) ccw projected
  arc A197 (166.9913, 125.787) -> (165.989, 125.1117) centre (170.2957, 119.8004) ccw projected
  arc A198 (165.989, 125.1117) -> (165.7382, 124.878) centre (167.5573, 123.1777) ccw projected
  line L48 (165.7382, 124.878) -> (165.2066, 124.2651) projected
  arc A199 (165.2066, 124.2651) -> (163.5643, 125.5748) centre (148.5, 105.0001) ccw projected
  line L49 (163.5643, 125.5748) -> (164.0436, 126.2295) projected
  arc A200 (164.0436, 126.2295) -> (164.2156, 126.5259) centre (161.9811, 127.6245) ccw projected
  arc A201 (164.2156, 126.5259) -> (164.6509, 127.6534) centre (158.0791, 129.5428) ccw projected
  arc A202 (164.6509, 127.6534) -> (165.0751, 130.0054) centre (153.3202, 130.9111) ccw projected
  arc A203 (165.0751, 130.0054) -> (163.8373, 130.7832) centre (148.5, 105.0001) ccw projected
  arc A204 (163.8373, 130.7832) -> (161.9022, 129.3805) centre (169.7535, 120.5853) ccw projected
  arc A205 (161.9022, 129.3805) -> (161.0752, 128.4992) centre (166.4559, 124.2793) ccw projected
  arc A206 (161.0752, 128.4992) -> (160.8828, 128.2155) centre (163.0346, 126.9626) ccw projected
  line L50 (160.8828, 128.2155) -> (160.5009, 127.4996) projected
  arc A207 (160.5009, 127.4996) -> (158.6083, 128.4111) centre (148.5, 105.0001) ccw projected
  line L51 (158.6083, 128.4111) -> (158.9299, 129.156) projected
  arc A208 (158.9299, 129.156) -> (159.0317, 129.4833) centre (156.6087, 130.0571) ccw projected
  arc A209 (159.0317, 129.4833) -> (159.2052, 130.6793) centre (152.3777, 131.0591) ccw projected
  arc A210 (159.2052, 130.6793) -> (159.0953, 133.0668) centre (147.4336, 131.334) ccw projected
  arc A211 (159.0953, 133.0668) -> (157.7155, 133.5497) centre (148.5, 105.0001) ccw projected
  arc A212 (157.7155, 133.5497) -> (156.141, 131.7515) centre (165.7526, 124.9239) ccw projected
  arc A213 (156.141, 131.7515) -> (155.5309, 130.7083) centre (161.7157, 127.7915) ccw projected
  arc A214 (155.5309, 130.7083) -> (155.4064, 130.3889) centre (157.7831, 129.6462) ccw projected
  line L52 (155.4064, 130.3889) -> (155.1934, 129.606) projected
  arc A215 (155.1934, 129.606) -> (153.1454, 130.0734) centre (148.5, 105.0001) ccw projected
  line L53 (153.1454, 130.0734) -> (153.2932, 130.8712) projected
  arc A216 (153.2932, 130.8712) -> (153.3196, 131.213) centre (150.8297, 131.2332) ccw projected
  arc A217 (153.3196, 131.213) -> (153.2226, 132.4176) centre (146.4818, 131.2686) ccw projected
  arc A218 (153.2226, 132.4176) -> (152.5843, 134.7208) centre (141.6005, 130.4365) ccw projected
  arc A219 (152.5843, 134.7208) -> (151.1315, 134.8845) centre (148.5, 105.0001) ccw projected
  arc A220 (151.1315, 134.8845) -> (149.9967, 132.7811) centre (160.8866, 128.2635) ccw projected
  arc A221 (149.9967, 132.7811) -> (149.6341, 131.6283) centre (156.3128, 130.1609) ccw projected
  arc A222 (149.6341, 131.6283) -> (149.5837, 131.2892) centre (152.0661, 131.0939) ccw projected
  line L54 (149.5837, 131.2892) -> (149.5503, 130.4785) projected
  arc A223 (149.5503, 130.4785) -> (147.4496, 130.4785) centre (148.5, 105.0001) ccw projected
  line L55 (147.4496, 130.4785) -> (147.4162, 131.2892) projected
  circle A224 centre (148.5, 105.0001) radius 21.5
  circle A225 centre (148.5, 105.0001) radius 8
  line L56 (147, 128.2635) -> (147, 81.1817)
  line L57 (150, 81.5011) -> (150, 128.2635)
  line L58 (125.8756, 106.5001) -> (171.1443, 106.5001)
  line L59 (172.6887, 103.5001) -> (124.6815, 103.5001)
  line L60 (145.7, 107.8001) -> (151.3, 107.8001) construction
  line L61 (151.3, 107.8001) -> (151.3, 102.2001) construction
  line L62 (151.3, 102.2001) -> (145.7, 102.2001) construction
  line L63 (145.7, 102.2001) -> (145.7, 107.8001) construction
  circle A226 centre (151.3, 107.8001) radius 1.5
  circle A227 centre (151.3, 102.2001) radius 1.5
  circle A228 centre (145.7, 102.2001) radius 1.5
  circle A229 centre (145.7, 107.8001) radius 1.5
  point P0 (0, 0)
  point P1 (169.9476, 103.5001)
  point P2 (156.3581, 103.5001)
  point P3 (150, 97.142)
  point P4 (150, 83.5525)
  point P5 (140.6418, 103.5001)
  point P6 (127.0524, 103.5001)
  point P7 (147, 83.5525)
  point P8 (147, 97.142)
  point P9 (127.0524, 106.5001)
  point P10 (140.6418, 106.5001)
  point P11 (147, 112.8583)
  point P12 (147, 126.4478)
  point P13 (156.3581, 106.5001)
  point P14 (169.9476, 106.5001)
  point P15 (150, 126.4478)
  point P16 (150, 112.8583)
  dimension "d4" = 4
  dimension "d6" = 1.5
  dimension "d7" = 3
  dimension "d8" = 1.5
  dimension "d9" = 3
  dimension "d17" = 5.6
  dimension "d18" = 3
  dimension "d19" = 3
  dimension "d20" = 3
  dimension "d21" = 3
  dimension "d22" = 16
  constraints: 16 end point, 7 coincident, 6 centre point, 3 horizontal, 2 vertical, 9 other
  measures "d4" radial gap between concentric circles of A223 A224
  measures "d6" distance from line of L57 A3.centre
  measures "d7" distance between parallel lines of L57 L56
  measures "d8" distance from line of L58 A3.centre
  measures "d9" distance between parallel lines of L58 L59
  measures "d17" distance of L60.end L61.end
  measures "d18" diameter of A226
  measures "d19" diameter of A227